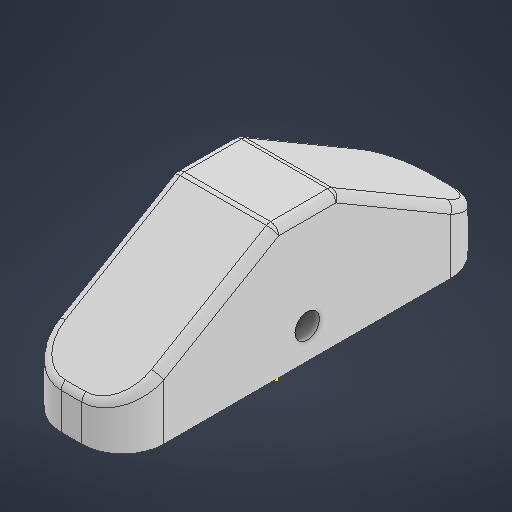
# Autodesk Inventor part: Triangle_Bracket
Saved by Autodesk Inventor 2026.2 (Build 302298000, 298)
## iProperties
Created: 2025-12-09
Part Number: Triangle_Bracket
Material: Generic
Document SubType Name: Modeling
Designer: Thoma
Density: 1 g/cm^3
Appearance: Default
Author: Thoma
Autodesk Inventor part; units mm, degrees
ref_plane "YZ Plane" through (0, 0, 0) normal (1, 0, 0) x (0, 1, 0)
ref_plane "XZ Plane" through (0, 0, 0) normal (0, 1, 0) x (-1, 0, 0)
ref_plane "XY Plane" through (0, 0, 0) normal (0, 0, 1) x (1, 0, 0)
sketch "Sketch1" plane through (0, 0, 0) normal (0, 1, 0) x (-1, 0, 0)
  line L0 (0, 0) -> (25, 0)
  line L1 (25, 0) -> (25, -90)
  line L2 (25, -90) -> (0, -90)
  line L3 (0, -90) -> (0, 0)
  dimension "d0" = 25
  dimension "d1" = 90
  constraints: 8 end point, 2 parallel, 1 horizontal, 1 perpendicular
  measures "d0" distance between parallel lines of L3 L1
  measures "d1" distance between parallel lines of L2 L0
extrude "Extrusion1" add sketch "Sketch1" along normal blind 10
sketch "Sketch2" plane through (0, 10, 0) normal (0, 1, 0) x (1, 0, 0)
  line L0 (-25, 90) -> (-25, 0) projected
  line L1 (0, 0) -> (0, 90) projected
  line L2 (-25, 37.5) -> (0, 37.5)
  line L3 (0, 37.5) -> (0, 52.5)
  line L4 (0, 52.5) -> (-25, 52.5)
  line L5 (-25, 52.5) -> (-25, 37.5)
  line L6 (-25, 0) -> (0, 0) projected
  point P0 (-25, 80)
  point P1 (-25, 10)
  point P2 (0, 10)
  point P3 (0, 80)
  point P4 (-15, 0)
  point P5 (-10, 0)
  point P6 (0, 37.5)
  dimension "d5" = 15
  dimension "d6" = 37.5
  constraints: 8 end point, 2 parallel, 2 point on line, 1 horizontal, 1 perpendicular
  measures "d5" distance between parallel lines of L4 L2
  measures "d6" distance between parallel lines of L6 L2
extrude "Extrusion2" add sketch "Sketch2" along normal blind 22 contours L4 L1 L2 L0
sketch "Sketch3" plane through (-25, 10, -37.5) normal (0, 0, 1) x (1, 0, 0)
  point P0 (25, -10)
sketch "Sketch5" plane through (0, 0, 0) normal (1, 0, 0) x (0, 0, -1)
  line L0 (37.5, 10) -> (37.5, 32) projected
  line L1 (0, 10) -> (37.5, 10) projected
  line L2 (37.5, 32) -> (0, 10)
  line L3 (37.5, 32) -> (52.5, 32) projected
  line L4 (52.5, 32) -> (90, 10)
  line L5 (90, 10) -> (52.5, 10) projected
  line L6 (52.5, 10) -> (90, 10)
  line L7 (52.5, 10) -> (52.5, 32) projected
  line L8 (52.5, 32) -> (52.5, 10)
  point P0 (0, 0)
  constraints: 8 end point, 2 collinear
extrude "Extrusion3" add sketch "Sketch5" against normal blind 25
fillet "Fillet2" radius 10 4 edges at (-25, 5, 0) (0, 5, 0) (-25, 5, -90) (0, 5, -90)
fillet "Fillet3" radius 2 14 edges at (-12.5, 32, -52.5) (-12.5, 32, -37.5) (0, 32, -45) (-2.9289, 11.7183, -87.0711) (-12.5, 10, -90) (-22.0711, 11.7183, -87.0711) (-25, 23.9333, -66.25) (0, 23.9333, -66.25) (-2.9289, 11.7183, -2.9289) (-12.5, 10, 0) (-22.0711, 11.7183, -2.9289) (-25, 23.9333, -23.75) (0, 23.9333, -23.75) (-25, 32, -45)
sketch "Sketch6" plane through (-25, 0, -80) normal (-1, 0, 0) x (0, 0, 1)
  line L0 (28.0434, 30) -> (41.9566, 30) projected
  line L1 (35, 30) -> (35, 15)
  line L2 (70, 0) -> (0, 0) projected
  line L3 (35, 30) -> (35, 0)
  line L4 (35, 15) -> (35, 0)
  circle A0 centre (35, 7.5) radius 3
  point P0 (80, 0)
  point P1 (35, 22.5)
  dimension "d13" = 6
  dimension "d14" = 7.5
  constraints: 6 end point, 5 midpoint, 2 collinear, 1 centre point
  measures "d13" diameter of A0
  measures "d14" distance of L1.end point (35, 22.5)
extrude "Extrusion4" cut sketch "Sketch6" against normal blind 25
sketch "Sketch7" plane through (-25, 0, -80) normal (-1, 0, 0) x (0, 0, 1)
  line L0 (35, 25.5581) -> (35, 19.5581)
  circle A0 centre (35, 7.5) radius 3 projected
  line L1 (35, 10.5) -> (35, 4.5)
  circle A1 centre (35, 7.5) radius 5
  point P0 (80, 0)
  point P1 (35, 22.5581)
  dimension "d19" = 10
  constraints: 4 end point, 2 point on circle, 1 centre point, 1 coincident, 1 vertical
  measures "d19" diameter of A1
extrude "Extrusion5" cut sketch "Sketch7" against normal blind 10
fillet "Fillet4" radius 1 1 edges at (-25, 7.5, -50)
sketch "Sketch8" plane through (0, 0, 0) normal (0, -1, 0) x (1, 0, 0)
  line L0 (-10, -90) -> (-15, -90) projected
  line L1 (-12.5, -90) -> (-12.5, 0)
  line L2 (-15, 0) -> (-10, 0) projected
  circle A0 centre (-12.5, -80.5935) radius 5
  circle A1 centre (-12.5, -9.4065) radius 5
  point P0 (0, 0)
  point P1 (-12.5, -45)
  point P2 (-12.5, -4.4065)
  point P3 (-12.5, -14.4065)
  point P4 (-12.5, -75.5935)
  point P5 (-12.5, -85.5935)
  dimension "d23" = 71.187
  dimension "d24" = 10
  dimension "d25" = 10
  dimension "d26" = 35.5935
  constraints: 3 midpoint, 2 centre point, 2 end point, 2 point on line
  measures "d23" distance of A1.centre A0.centre
  measures "d24" diameter of A0
  measures "d25" diameter of A1
  measures "d26" distance of A0.centre point (-12.5, -45)
extrude "Extrusion6" cut sketch "Sketch8" against normal blind 10
body "Solid1"
